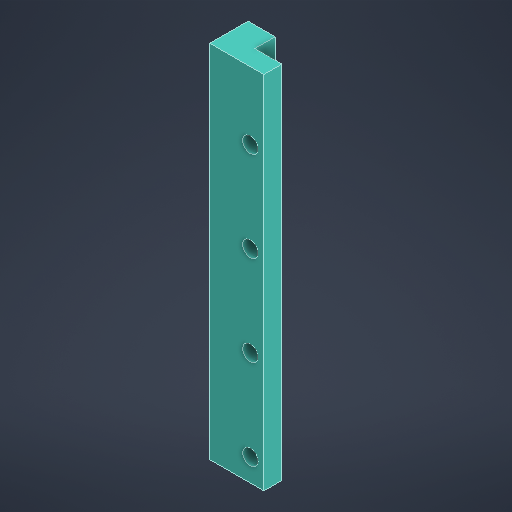
# Autodesk Inventor part: Right_Rod_Support
Saved by Autodesk Inventor 2027.1 (Build 311270010, 270A)
## iProperties
Created: 2026-09-22
Part Number: Right_Rod_Support
Material: Generic
Document SubType Name: Modeling
Designer: 박정현
Density: 1 g/cm^3
Appearance: Right separate support; four original rod clearance holes and four blind M3 x 0.5 - 6H deck threads, 6.5 mm depth.
Author: 박정현
Comments: Right separate support; four original rod clearance holes and four blind M3 x 0.5 - 6H deck threads, 6.5 mm depth.
Autodesk Inventor part; units mm, degrees
ref_plane "Right_Connecting_Web_StartPlane" through (0, 0, 4) normal (0, 0, 1) x (1, 0, 0)
sketch "Right_Connecting_Web_Profile" plane through (0, 0, 4) normal (0, 0, 1) x (1, 0, 0)
  line L0 (39, 0) -> (45, 0)
  line L1 (45, 0) -> (45, 80)
  line L2 (45, 80) -> (39, 80)
  line L3 (39, 80) -> (39, 0)
  point P0 (0, 0)
  dimension "d1" = 39
  dimension "d2" = 6
  dimension "d3" = 80
  constraints: 8 end point, 2 parallel, 1 horizontal, 1 horizontal alignment, 1 perpendicular
  measures "d1" distance of point (0, 0) L0.start
  measures "d2" distance of L1.end L2.end
  measures "d3" distance of L2.end L0.start
extrude "Right_Connecting_Web" add sketch "Right_Connecting_Web_Profile" along normal blind 8.5
ref_plane "Right_Rod_Contact_Flange_StartPlane" through (0, 0, 8.5) normal (0, 0, 1) x (1, 0, 0)
sketch "Right_Rod_Contact_Flange_Profile" plane through (0, 0, 8.5) normal (0, 0, 1) x (1, 0, 0)
  line L0 (39, 0) -> (51, 0)
  line L1 (51, 0) -> (51, 80)
  line L2 (51, 80) -> (39, 80)
  line L3 (39, 80) -> (39, 0)
  point P0 (0, 0)
  dimension "d7" = 39
  dimension "d8" = 12
  dimension "d9" = 80
  constraints: 8 end point, 2 parallel, 1 horizontal, 1 horizontal alignment, 1 perpendicular
  measures "d7" distance of point (0, 0) L0.start
  measures "d8" distance of L1.end L2.end
  measures "d9" distance of L2.end L0.start
extrude "Right_Rod_Contact_Flange" add sketch "Right_Rod_Contact_Flange_Profile" along normal blind 4
sketch "Original_Rod_Clearance_4x_Locations" plane through (0, 0, 0) normal (0, 0, 1) x (1, 0, 0)
  circle A0 centre (48, 5) radius 1.7
  circle A1 centre (48, 25) radius 1.7
  circle A2 centre (48, 45) radius 1.7
  circle A3 centre (48, 65) radius 1.7
  point P0 (0, 0)
  dimension "d12" = 48
  dimension "d13" = 5
  dimension "d14" = 3.4
  dimension "d15" = 48
  dimension "d16" = 25
  dimension "d17" = 3.4
  dimension "d18" = 48
  dimension "d19" = 45
  dimension "d20" = 3.4
  dimension "d21" = 48
  dimension "d22" = 65
  dimension "d23" = 3.4
  constraints: 4 centre point
  measures "d12" horizontal distance of point (0, 0) A0.centre
  measures "d13" vertical distance of point (0, 0) A0.centre
  measures "d14" diameter of A0
  measures "d15" horizontal distance of point (0, 0) A1.centre
  measures "d16" vertical distance of point (0, 0) A1.centre
  measures "d17" diameter of A1
  measures "d18" horizontal distance of point (0, 0) A2.centre
  measures "d19" vertical distance of point (0, 0) A2.centre
  measures "d20" diameter of A2
  measures "d21" horizontal distance of point (0, 0) A3.centre
  measures "d22" vertical distance of point (0, 0) A3.centre
  measures "d23" diameter of A3
extrude "Original_Rod_Clearance_4x" cut sketch "Original_Rod_Clearance_4x_Locations" along normal through all
ref_plane "Work Plane3" through (0, 0, 4) normal (0, 0, 1) x (1, 0, 0)
sketch "Deck_Assembly_M3_Locations" plane through (0, 0, 4) normal (0, 0, 1) x (1, 0, 0)
  circle A0 centre (41.5, 10) radius 1.25
  circle A1 centre (41.5, 30) radius 1.25
  circle A2 centre (41.5, 50) radius 1.25
  circle A3 centre (41.5, 70) radius 1.25
  point P0 (0, 0)
  dimension "d27" = 41.5
  dimension "d28" = 10
  dimension "d29" = 2.5
  dimension "d30" = 41.5
  dimension "d31" = 30
  dimension "d32" = 2.5
  dimension "d33" = 41.5
  dimension "d34" = 50
  dimension "d35" = 2.5
  dimension "d36" = 41.5
  dimension "d37" = 70
  dimension "d38" = 2.5
  constraints: 4 centre point
  measures "d27" horizontal distance of point (0, 0) A0.centre
  measures "d28" vertical distance of point (0, 0) A0.centre
  measures "d29" diameter of A0
  measures "d30" horizontal distance of point (0, 0) A1.centre
  measures "d31" vertical distance of point (0, 0) A1.centre
  measures "d32" diameter of A1
  measures "d33" horizontal distance of point (0, 0) A2.centre
  measures "d34" vertical distance of point (0, 0) A2.centre
  measures "d35" diameter of A2
  measures "d36" horizontal distance of point (0, 0) A3.centre
  measures "d37" vertical distance of point (0, 0) A3.centre
  measures "d38" diameter of A3
extrude "Four_Blind_M3_Tap_Bores" cut sketch "Deck_Assembly_M3_Locations" along normal blind 6.5
thread "Deck_M3x0_5_6H_1" size "M3x0.5" class "6H" standard "ISO Metric profile" length 6.5
thread "Deck_M3x0_5_6H_2" size "M3x0.5" class "6H" standard "ISO Metric profile" length 6.5
thread "Deck_M3x0_5_6H_3" size "M3x0.5" class "6H" standard "ISO Metric profile" length 6.5
thread "Deck_M3x0_5_6H_4" size "M3x0.5" class "6H" standard "ISO Metric profile" length 6.5
equation "\"d1\" = -RodWidth + OverallWidth - WebThickness"
equation "\"d2\" = WebThickness"
equation "\"d3\" = ContactLength"
equation "\"d4\" = DropHeight"
equation "\"d7\" = -RodWidth + OverallWidth - WebThickness"
equation "\"d8\" = RodWidth + WebThickness"
equation "\"d9\" = ContactLength"
equation "\"d10\" = BaseThickness"
equation "\"d12\" = OverallWidth - 0.5 * RodWidth"
equation "\"d13\" = RodHoleStart + 0 * RodScrewPitch"
equation "\"d14\" = RodClearanceDiameter"
equation "\"d15\" = OverallWidth - 0.5 * RodWidth"
equation "\"d16\" = RodHoleStart + RodScrewPitch"
equation "\"d17\" = RodClearanceDiameter"
equation "\"d18\" = OverallWidth - 0.5 * RodWidth"
equation "\"d19\" = RodHoleStart + 2 * RodScrewPitch"
equation "\"d20\" = RodClearanceDiameter"
equation "\"d21\" = OverallWidth - 0.5 * RodWidth"
equation "\"d22\" = RodHoleStart + 3 * RodScrewPitch"
equation "\"d23\" = RodClearanceDiameter"
equation "\"d27\" = OverallWidth - JoinLeftX"
equation "\"d28\" = JoinFirstY + 0 * JoinPitch"
equation "\"d29\" = TapDrillDiameter"
equation "\"d30\" = OverallWidth - JoinLeftX"
equation "\"d31\" = JoinFirstY + JoinPitch"
equation "\"d32\" = TapDrillDiameter"
equation "\"d33\" = OverallWidth - JoinLeftX"
equation "\"d34\" = JoinFirstY + 2 * JoinPitch"
equation "\"d35\" = TapDrillDiameter"
equation "\"d36\" = OverallWidth - JoinLeftX"
equation "\"d37\" = JoinFirstY + 3 * JoinPitch"
equation "\"d38\" = TapDrillDiameter"
equation "\"d39\" = JoinThreadDepth"
equation "\"d41\" = JoinThreadDepth"
equation "\"d43\" = JoinThreadDepth"
equation "\"d45\" = JoinThreadDepth"
equation "\"d47\" = JoinThreadDepth"
equation "\"OverallWidth\" = 51"
equation "\"RodWidth\" = 6"
equation "\"ContactLength\" = 80"
equation "\"BaseThickness\" = 4"
equation "\"DropHeight\" = 8.5"
equation "\"WebThickness\" = 6"
equation "\"FingerStartX\" = 19.93338"
equation "\"FingerWidth\" = 13.5"
equation "\"FingerThickness\" = 6"
equation "\"FingerEndInset\" = 4"
equation "\"RodClearanceDiameter\" = 3.4"
equation "\"ClampFirstY\" = 41.82802"
equation "\"ClampPitch\" = 16"
equation "\"ClampHeight\" = BaseThickness + 0.5 * FingerThickness"
equation "\"TapDrillDiameter\" = 2.5"
equation "\"TapDepth\" = 6"
equation "\"RodHoleStart\" = 5"
equation "\"RodScrewPitch\" = 20"
equation "\"JoinLeftX\" = 9.5"
equation "\"JoinFirstY\" = 10"
equation "\"JoinPitch\" = 20"
equation "\"JoinThreadDepth\" = 6.5"
equation "\"JoinCountersinkDiameter\" = 6.2"
equation "\"d0\" = BaseThickness"
equation "\"d6\" = DropHeight"
equation "\"d26\" = BaseThickness"
body "Solid1"
